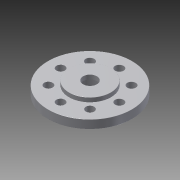
# Autodesk Inventor part: Low_Height_Horn
Saved by Autodesk Inventor 2013 (Build 170138000, 138)
## iProperties
Created: 2014-01-06
Material: アセタール樹脂、白
Document SubType Name: Modeling
Designer: andou
Density: 1.425 g/cm^3
Mass: 0.914321 g
Surface Area: 9.1177 cm^2
Volume: 0.641628 cm^3
Author: andou
Title: Low_Height_Horn
Autodesk Inventor part; units mm, degrees
ref_plane "YZ Plane" through (0, 0, 0) normal (1, 0, 0) x (0, 1, 0)
ref_plane "XZ Plane" through (0, 0, 0) normal (0, 1, 0) x (-1, 0, 0)
ref_plane "XY Plane" through (0, 0, 0) normal (0, 0, 1) x (1, 0, 0)
sketch "スケッチ1" plane through (0, 0, 0) normal (0, 0, 1) x (1, 0, 0)
  circle A0 centre (0, 0) radius 10
  dimension "d0" = 20
  constraints: 1 centre point, 1 coincident
  measures "d0" diameter of A0
extrude "押し出し1" add sketch "スケッチ1" along normal blind 2
sketch "スケッチ2" plane through (0, 0, 2) normal (0, 0, 1) x (1, 0, 0)
  circle A0 centre (0, 0) radius 10 projected
  circle A1 centre (0, 0) radius 5
  dimension "d3" = 10
  constraints: 1 centre point, 1 coincident
  measures "d3" diameter of A1
extrude "押し出し2" add sketch "スケッチ2" along normal blind 1 contours A1
sketch "スケッチ4" plane through (0, 0, 0) normal (0, 0, -1) x (-1, 0, 0)
  circle A0 centre (0, 0) radius 10 projected
  circle A1 centre (0, 0) radius 5
  dimension "d6" = 10
  constraints: 1 centre point, 1 coincident
  measures "d6" diameter of A1
extrude "押し出し3" add sketch "スケッチ4" along normal blind 1 contours A1
sketch "スケッチ5" plane through (0, 0, -1) normal (0, 0, -1) x (-1, 0, 0)
  circle A0 centre (0, 0) radius 5 projected
  circle A1 centre (0, 0) radius 3
  dimension "d9" = 6
  constraints: 1 centre point, 1 coincident
  measures "d9" diameter of A1
extrude "押し出し4" cut sketch "スケッチ5" against normal blind 3 contours A1
sketch "スケッチ6" plane through (0, 0, 2) normal (0, 0, -1) x (-1, 0, 0)
  circle A0 centre (0, 0) radius 3 projected
  circle A1 centre (0, 0) radius 1.65
  dimension "d12" = 3.3
  constraints: 1 centre point, 1 coincident
  measures "d12" diameter of A1
hole "穴1" at (0, 0, 2) direction (0, 0, 1) diameter 3.3 end through all
sketch "スケッチ7" plane through (0, 0, 0) normal (0, 0, -1) x (-1, 0, 0)
  circle A0 centre (0, 0) radius 5 projected
  circle A1 centre (-7, 0) radius 1
  dimension "d20" = 2
  dimension "d21" = 7
  constraints: 1 centre point
  measures "d20" diameter of A1
  measures "d21" distance of A0.centre A1.centre
hole "穴2" at (7, 0, 0) direction (0, 0, 1) diameter 2 end through all
pattern_circular "円形状パターン1" count 8 over 360 about axis through (0, 0, -1) along (0, 0, 1) of "穴2"
fillet "フィレット3" radius 0.05 12 edges at (-10, 0, 2) (-10, 0, 0) (1, 7, 2) (5.6569, 4.2426, 2) (7, -1, 2) (-4.2426, 5.6569, 2) (-4.2426, 5.6569, 0) (7, -1, 0) (5.6569, 4.2426, 0) (1, 7, 0) (5, 0, -1) (-5, 0, 3)
